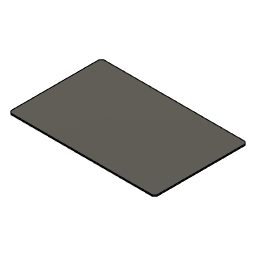
Play_Base (Autodesk Fusion 360 design; units mm, degrees)
Autodesk Fusion 360 part; units mm, degrees
sketch "Sketch1" plane through (0, 0, 0) normal (0, 0, 1) x (1, 0, 0)
  line L0 (-835.025, 530.225) -> (835.025, 530.225)
  line L1 (835.025, 530.225) -> (835.025, -530.225)
  line L2 (835.025, -530.225) -> (-835.025, -530.225)
  line L3 (-835.025, -530.225) -> (-835.025, 530.225)
  line L4 (-835.025, 530.225) -> (835.025, -530.225) construction
  line L5 (835.025, 530.225) -> (-835.025, -530.225) construction
  dimension "d1" = 1670.05
  dimension "d2" = 1060.45
  constraint horizontal L0
  constraint perpendicular L0 L1
  constraint parallel L0 L2
  constraint parallel L1 L3
  constraint coincident L4 origin
  constraint coincident L5 origin
  measures "d1" distance of L0.start L0.end
  measures "d2" distance of L0.end L1.end
extrude "Extrude1" add sketch "Sketch1" along normal blind 12.7
chamfer "Chamfer1" distance 25.4 angle 45 4 edges at (-835.025, -530.225, 6.35) (-835.025, 530.225, 6.35) (835.025, 530.225, 6.35) (835.025, -530.225, 6.35)
equation "d1 = 66 in - 0.25 in"
equation "d2 = 42 in - 0.25 in"
